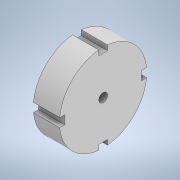
# Autodesk Inventor part: 711143
Saved by Autodesk Inventor 2022 (Build 260153000, 153)
## iProperties
Created: 2021-10-22
Part Number: 711143
Material: Типовые
Document SubType Name: Modeling
Designer: RaNSiD
Density: 1 g/cm^3
Appearance: По умолчанию
Author: RaNSiD
Autodesk Inventor part; units mm, degrees
ref_plane "YZ Plane" through (0, 0, 0) normal (1, 0, 0) x (0, 1, 0)
ref_plane "XZ Plane" through (0, 0, 0) normal (0, 1, 0) x (-1, 0, 0)
ref_plane "XY Plane" through (0, 0, 0) normal (0, 0, 1) x (1, 0, 0)
sketch "Эскиз1" plane through (0, 0, 0) normal (0, 0, 1) x (1, 0, 0)
  line L0 (0, 0) -> (15, 0)
  line L1 (15, 0) -> (15, 25)
  line L2 (15, 25) -> (0, 25)
  line L3 (0, 25) -> (0, 0)
  dimension "d0" = 15
  dimension "d1" = 25
  constraints: 8 end point, 2 parallel, 1 horizontal, 1 perpendicular
  measures "d0" distance of L2.end L1.end
  measures "d1" distance of L1.end L0.end
revolve "Вращение1" add sketch "Эскиз1" angle 360 about axis through (0, 0, 0) along (1, 0, 0)
sketch "Эскиз2" plane through (0, 0, 0) normal (-1, 0, 0) x (0, 0, 1)
  circle A0 centre (0, 0) radius 2.5
  line L0 (22, 2.5) -> (22, -2.5)
  line L1 (22, -2.5) -> (24.8747, -2.5)
  circle A1 centre (0, 0) radius 25 projected
  line L2 (24.8747, 2.5) -> (22, 2.5)
  arc A2 (24.8747, -2.5) -> (24.8747, 2.5) centre (0, 0) ccw
  line L3 (-2.5, 24.8747) -> (-2.5, 22)
  line L4 (2.5, 22) -> (2.5, 24.8747)
  line L5 (-2.5, 22) -> (2.5, 22)
  arc A3 (2.5, 24.8747) -> (-2.5, 24.8747) centre (0, 0) ccw
  line L6 (-24.8747, -2.5) -> (-22, -2.5)
  line L7 (-22, 2.5) -> (-24.8747, 2.5)
  line L8 (-22, -2.5) -> (-22, 2.5)
  arc A4 (-24.8747, 2.5) -> (-24.8747, -2.5) centre (0, 0) ccw
  line L9 (2.5, -24.8747) -> (2.5, -22)
  line L10 (-2.5, -22) -> (-2.5, -24.8747)
  line L11 (2.5, -22) -> (-2.5, -22)
  arc A5 (-2.5, -24.8747) -> (2.5, -24.8747) centre (0, 0) ccw
  point P0 (22, 0)
  point P1 (25, 0)
  point P2 (0, 22)
  point P3 (0, 25)
  point P4 (-22, 0)
  point P5 (-25, 0)
  point P6 (0, -22)
  point P7 (0, -25)
  dimension "d3" = 5
  dimension "d4" = 5
  dimension "d5" = 22
  dimension "d8" = 360
  constraints: 24 end point, 12 point on circle, 5 centre point, 3 coincident, 2 horizontal alignment, 1 horizontal, 1 midpoint, 1 parallel, 1 perpendicular, 43 other
  measures "d3" diameter of A0
  measures "d4" distance of L0.start L0.end
  measures "d5" distance of point (0, 0) point (22, 0)
extrude "Выдавливание1" cut sketch "Эскиз2" against normal through all contours A0 | L2 A1 L1 L0 | L4 L5 L3 A1 | A1 L10 L11 L9 | L7 L8 L6 A1
